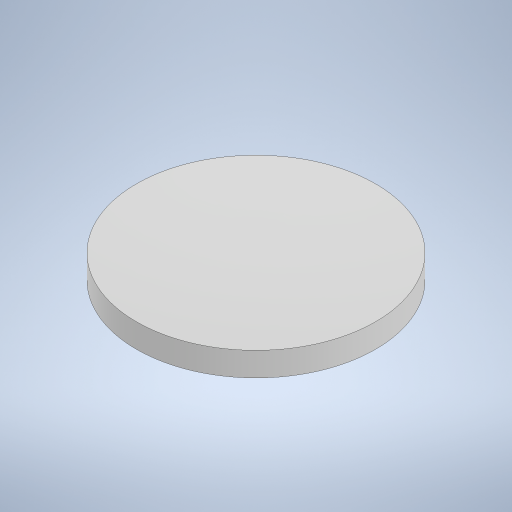
# Autodesk Inventor part: зрачок
Saved by Autodesk Inventor 2023.2 (Build 272271030, 271C)
## iProperties
Created: 2024-03-18
Part Number: зрачок
Material: Типовые
Document SubType Name: Modeling
Designer: I9232
Density: 1 g/cm^3
Appearance: По умолчанию
Author: I9232
Autodesk Inventor part; units mm, degrees
ref_plane "YZ Plane" through (0, 0, 0) normal (1, 0, 0) x (0, 1, 0)
ref_plane "XZ Plane" through (0, 0, 0) normal (0, 1, 0) x (-1, 0, 0)
ref_plane "XY Plane" through (0, 0, 0) normal (0, 0, 1) x (1, 0, 0)
sketch "Эскиз1" plane through (0, 0, 0) normal (0, 0, 1) x (1, 0, 0)
  line L0 (-15, 0) -> (-15, 3)
  line L1 (-15, 0) -> (0, 0)
  line L2 (0, 2.3791) -> (0, 0.5542) construction
  arc A0 (0, 5.3) -> (-15, 3) centre (0, -44.763) ccw
  line L3 (0, 0) -> (0, 5.3) construction
  line L4 (0, 5.3) -> (0, 0)
  dimension "d0" = 3
  dimension "d1" = 15
  dimension "d6" = 5.3
  constraints: 10 end point, 3 vertical, 2 point on circle, 1 centre point, 1 horizontal, 1 line through centre, 1 perpendicular
  measures "d0" distance of L0.start L0.end
  measures "d1" distance of L0.start L1.end
  measures "d6" distance from line of L1 L3.end
revolve "Вращение1" add sketch "Эскиз1" angle 360 about axis through (0, 5.3, 0) along (0, -1, 0)
shell "Оболочка1" thickness 0.5 removed faces 1 at (-4.7094, 0, 0) ; own thickness 0.25 on faces at (-14.9514, 2, 1.207)
fillet "Сопряжение1" radius 1 1 edges at (14.75, 2.5543, 0.0003)
